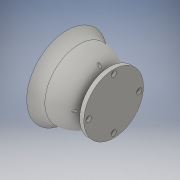
# Autodesk Inventor part: Launcher Cup
Saved by Autodesk Inventor 2016 (Build 200138000, 138)
## iProperties
Created: 2016-11-08
Part Number: Launcher Cup
Material: Generic
Document SubType Name: Modeling
Designer: paul_
Density: 1 g/cm^3
Appearance: Default
Author: paul_
Autodesk Inventor part; units mm, degrees
ref_plane "YZ Plane" through (0, 0, 0) normal (1, 0, 0) x (0, 1, 0)
ref_plane "XZ Plane" through (0, 0, 0) normal (0, 1, 0) x (-1, 0, 0)
ref_plane "XY Plane" through (0, 0, 0) normal (0, 0, 1) x (1, 0, 0)
sketch "Sketch1" plane through (0, 0, 0) normal (0, 1, 0) x (-1, 0, 0)
  arc A0 (-48.26, 0) -> (-2.8901, -48.1734) centre (0, 0) ccw
  line L0 (0, 0) -> (2.3486, 0) construction
  arc A1 (-48.26, -15.8623) -> (-2.7486, -50.7256) centre (0, 0) ccw
  arc A2 (15.4672, -59.6495) -> (-2.7486, -50.7256) centre (-4.1531, -76.6458) ccw
  arc A3 (14.9178, -55.5155) -> (-2.8901, -48.1734) centre (-4.6642, -77.7436) ccw
  arc A4 (15.4672, -59.6495) -> (14.9178, -55.5155) centre (12.8191, -57.8979) ccw
  line L1 (31.2133, 0) -> (-72.6552, 0) projected
  line L2 (-48.26, 0) -> (-54.61, 0)
  line L3 (-54.61, 0) -> (-54.61, -44.45)
  line L4 (-54.61, -44.45) -> (-48.26, -44.45)
  line L5 (-48.26, -44.45) -> (-48.26, -15.8623)
  point P0 (-50.8, 0)
  dimension "d0" = 48.26
  dimension "d2" = 2.54
  dimension "d3" = 3.175
  dimension "d13" = 6.35
  dimension "d14" = 44.45
  dimension "d15" = 25.9583
  dimension "d16" = 29.6234
  dimension "d17" = 59.6495
  dimension "d18" = 55.5155
  dimension "d19" = 57.8979
  dimension "d20" = 50.6086
  dimension "d21" = 2.54
  constraints: 10 end point, 10 point on circle, 5 centre point, 4 tangent, 2 horizontal, 2 parallel, 2 point on line, 1 coincident, 1 perpendicular
  measures "d0" radius of A0
  measures "d2" radial gap between concentric circles of A0 A1
  measures "d3" radius of A4
  measures "d13" distance of L4.end L3.end
  measures "d14" distance of L3.end L2.end
  measures "d15" radius of A2
  measures "d16" radius of A3
  measures "d17" distance from line of A2.start L1
  measures "d18" distance from line of A3.start L1
  measures "d19" distance from line of A4.centre L1
  measures "d20" distance from line of L0.end L5
  measures "d21" distance from line of point (-50.8, 0) L5
revolve "Revolution1" add sketch "Sketch1" angle 360 about axis through (-10, 0, 0) along (1, 0, 0)
hole "Hole1" at (54.61, -2.8557, -38.0756) direction (-1, 0, 0) diameter 4.4958 end through all counterbore diameter 7.9502 counterbore depth 4.1656
hole "Hole2" at (54.61, -1.0655, 37.4744) direction (-1, 0, 0) diameter 4.4958 end through all counterbore diameter 7.9502 counterbore depth 4.1656
hole "Hole3" at (54.61, -37.5872, 0.0574) direction (-1, 0, 0) diameter 4.4958 end through all counterbore diameter 7.9502 counterbore depth 4.1656
hole "Hole4" at (54.61, 38.4998, -0.1216) direction (-1, 0, 0) diameter 4.4958 end through all counterbore diameter 7.9502 counterbore depth 4.1656
body "Solid1"
